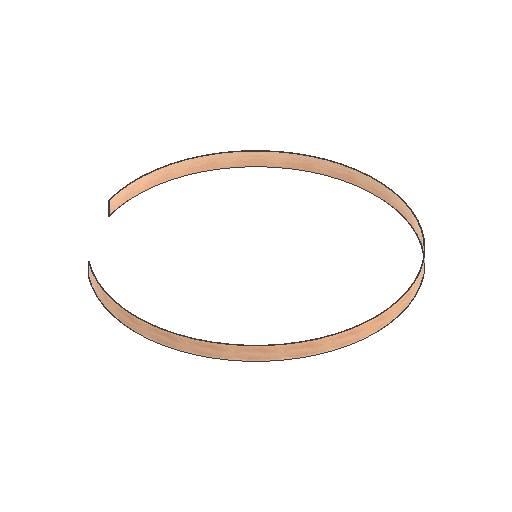
# Autodesk Inventor part: Edge Band - Platform C Inner
Saved by Autodesk Inventor 2021 (Build 250183000, 183)
## iProperties
Created: 2020-05-12
Part Number: Edge Band - Platform C Inner
Material: Wood (Birch)
Document SubType Name: Modeling
Designer: Dan Wikman
Density: 0.55 g/cm^3
Appearance: Birch - Natural Polished
Mass: 1089.93 g
Surface Area: 10313 cm^2
Volume: 1981.69 cm^3
Author: Dan Wikman
Autodesk Inventor part; units mm, degrees
ref_plane "YZ Plane" through (0, 0, 0) normal (1, 0, 0) x (0, 1, 0)
ref_plane "XZ Plane" through (0, 0, 0) normal (0, 1, 0) x (-1, 0, 0)
ref_plane "XY Plane" through (0, 0, 0) normal (0, 0, 1) x (1, 0, 0)
sketch "Sketch1" plane through (0, 0, 0) normal (0, 1, 0) x (-1, 0, 0)
  circle A0 centre (0, 0) radius 880.76
  circle A1 centre (0, 0) radius 876.76
  dimension "d0" = 1761.52
  dimension "d1" = 1753.52
  constraints: 2 centre point, 2 coincident
  measures "d0" diameter of A0
  measures "d1" diameter of A1
extrude "Extrusion1" add sketch "Sketch1" along normal blind 100
sketch "Sketch2" plane through (0, 100, 0) normal (0, 1, 0) x (1, 0, 0)
  line L0 (-1152.0023, -397.8039) -> (-847.3816, -240.1766) projected
  line L1 (-532.5688, -700.65) -> (-790.0008, -927.2838) projected
  circle A0 centre (0, 0) radius 876.76 projected
  line L2 (-530.0269, -698.4122) -> (-533.0898, -701.1087)
  circle A1 centre (0, 0) radius 880.76 projected
  line L3 (-847.3816, -240.1766) -> (-843.7518, -238.2983)
  point P0 (-843.7543, -238.2996)
  point P1 (-847.3805, -240.176)
  constraints: 4 end point, 1 point on line, 4 other
extrude "Extrusion2" cut sketch "Sketch2" against normal blind 100 contours L1 A1 L3 A0 L2 picked at (-840.9977, -251.8211)
body "Solid1"
